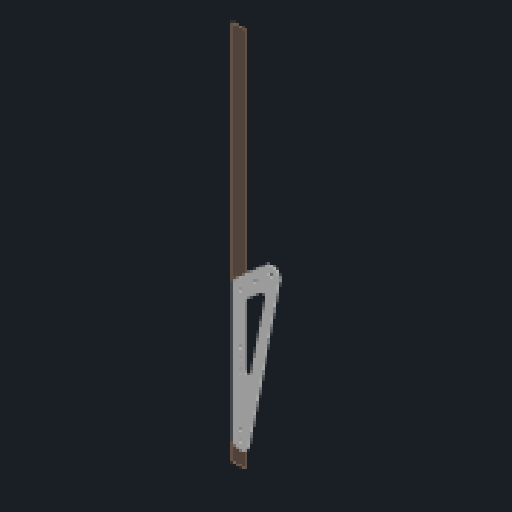
# Autodesk Inventor part: Part3
Saved by Autodesk Inventor 2025 (Build 290162010, 162A)
## iProperties
Created: 2025-11-04
Part Number: Part3
Material: Generic
Document SubType Name: Modeling
Designer: jasper
Density: 1 g/cm^3
Appearance: Default
Author: jasper
Autodesk Inventor part; units mm, degrees
ref_plane "YZ Plane" through (0, 0, 0) normal (1, 0, 0) x (0, 1, 0)
ref_plane "XZ Plane" through (0, 0, 0) normal (0, 1, 0) x (-1, 0, 0)
ref_plane "XY Plane" through (0, 0, 0) normal (0, 0, 1) x (1, 0, 0)
ref_plane "Work Plane1" through (0, 0, 0) normal (0, 0, 1) x (1, 0, 0)
sketch "Sketch1" plane through (0, 0, 0) normal (0, 0, 1) x (1, 0, 0)
  circle A0 centre (12.7, -209.55) radius 2.1844 projected
  circle A1 centre (12.7, -196.85) radius 2.1844 projected
  circle A2 centre (12.7, -133.35) radius 2.1844 projected
  circle A3 centre (12.7, -120.65) radius 2.1844 projected
  circle A4 centre (12.7, -107.95) radius 2.1844 projected
  circle A5 centre (12.7, -44.45) radius 2.1844 projected
  circle A6 centre (31.6579, -27.5456) radius 2.1844 projected
  circle A7 centre (50.6158, -10.6412) radius 2.1844 projected
  line L0 (2.3114, 215.9) -> (2.3114, -215.9) construction
  circle A8 centre (12.7, -209.55) radius 10.3886
  circle A9 centre (12.7, -44.45) radius 10.3886
  circle A10 centre (50.6158, -10.6412) radius 10.3886
  line L1 (60.8206, -12.5864) -> (22.9049, -211.4952)
  line L2 (2.3114, -209.55) -> (2.3114, -44.45)
  line L3 (43.7019, -2.8874) -> (5.7861, -36.6962)
  line L4 (48.3453, -10.2084) -> (10.4295, -209.1172)
  line L5 (21.59, -208.514) -> (21.59, -43.414)
  line L6 (57.5635, -18.4329) -> (18.0129, -53.6994)
  line L7 (19.05, -39.0398) -> (19.05, -100.5078) projected
  point P0 (0, 0)
  point P1 (21.59, -150.5683)
  point P2 (21.59, -50.5098)
  point P3 (44.5688, -30.02)
  dimension "d0" = 20.7772
  dimension "d1" = 20.7772
  dimension "d2" = 20.828
  dimension "d3" = 12.7
  dimension "d8" = 2.54
  constraints: 12 end point, 6 point on circle, 5 tangent, 3 centre point, 3 coincident, 3 parallel, 2 point on line
  measures "d0" diameter of A9
  measures "d1" diameter of A10
  measures "d2" distance between parallel lines of L6 L3
  measures "d3" distance between parallel lines of L1 L4
  measures "d8" distance between parallel lines of L5 L7
extrude "Extrusion1" add sketch "Sketch1" along normal blind 1.5875 contours A1 L4 L5 A8 | A1 L4 A8 L2 A9 L7 L6 L5 | L4 A10 L1 A8 L5 | A8 | L6 L5 A9 L3 A10 L4 | L6 L7 A9 L5 | A10 | A9
fillet "Fillet1" radius 3.175 3 edges at (21.59, -150.5683, 0.7937) (21.59, -50.5098, 0.7937) (44.5688, -30.02, 0.7937)
body "Solid1"
